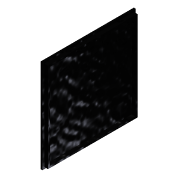
# Autodesk Inventor part: Zadní kryt
Saved by Autodesk Inventor 2015 (Build 190159000, 159)
## iProperties
Created: 2015-01-09
Part Number: Zadní kryt
Material: Všeobecné
Document SubType Name: Modeling
Designer: Michal
Density: 1 g/cm^3
Appearance: Černý
Author: Michal
Autodesk Inventor part; units mm, degrees
ref_plane "YZ Plane" through (0, 0, 0) normal (1, 0, 0) x (0, 1, 0)
ref_plane "XZ Plane" through (0, 0, 0) normal (0, 1, 0) x (-1, 0, 0)
ref_plane "XY Plane" through (0, 0, 0) normal (0, 0, 1) x (1, 0, 0)
sketch "Náčrt1" plane through (0, 0, 0) normal (1, 0, 0) x (0, 1, 0)
  line L0 (0, 0) -> (100, 0)
  line L1 (100, 0) -> (100, -100)
  line L2 (100, -100) -> (0, -100)
  line L3 (0, -100) -> (0, 0)
  dimension "d0" = 100
  dimension "d1" = 100
  constraints: 8 end point, 2 parallel, 1 horizontal, 1 perpendicular
  measures "d0" distance of L1.end L2.end
  measures "d1" distance of L0.end L1.end
extrude "Vysunutí1" add sketch "Náčrt1" along normal blind 2
sketch "Náčrt2" plane through (2, 0, 0) normal (1, 0, 0) x (0, 0, -1)
  line L0 (0, 100) -> (0, 0) projected
  line L1 (0, 0) -> (100, 0) projected
  line L2 (100, 0) -> (100, 100) projected
  line L3 (100, 100) -> (0, 100) projected
  line L4 (2, 98) -> (2, 2)
  line L5 (2, 2) -> (98, 2)
  line L6 (98, 2) -> (98, 98)
  line L7 (98, 98) -> (2, 98)
  line L8 (4, 96) -> (4, 4)
  line L9 (4, 4) -> (96, 4)
  line L10 (96, 4) -> (96, 96)
  line L11 (96, 96) -> (4, 96)
  dimension "d4" = 2
  dimension "d5" = 2
  constraints: 16 end point, 6 other
  measures "d4" distance between parallel lines of L3 L7
  measures "d5" distance between parallel lines of L7 L11
extrude "Vysunutí2" add sketch "Náčrt2" along normal blind 4 contours L7 L6 L5 L4
